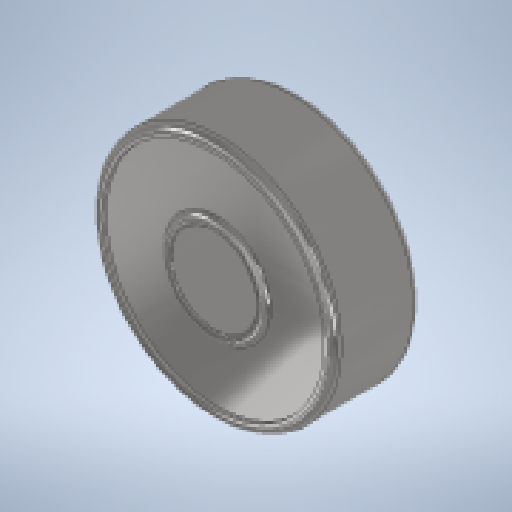
# Autodesk Inventor part: Bearing_small
Saved by Autodesk Inventor 2024 (Build 280153000, 153)
## iProperties
Created: 2025-02-20
Part Number: Bearing_small
Material: 一般
Document SubType Name: Modeling
Designer: tanoue_kota
Density: 1 g/cm^3
Appearance: 鋼 - つや出し
Author: tanoue_kota
Autodesk Inventor part; units mm, degrees
ref_plane "YZ Plane" through (0, 0, 0) normal (1, 0, 0) x (0, 1, 0)
ref_plane "XZ Plane" through (0, 0, 0) normal (0, 1, 0) x (-1, 0, 0)
ref_plane "XY Plane" through (0, 0, 0) normal (0, 0, 1) x (1, 0, 0)
sketch "スケッチ1" plane through (0, 0, 0) normal (0, 0, 1) x (1, 0, 0)
  circle A0 centre (0, 0) radius 8.5
  circle A1 centre (0, 0) radius 3
  dimension "d0" = 17
  dimension "d1" = 6
  constraints: 2 centre point, 2 coincident
  measures "d0" diameter of A0
  measures "d1" diameter of A1
extrude "押し出し1" add sketch "スケッチ1" along normal blind 3
sketch "スケッチ2" plane through (0, 0, 3) normal (0, 0, 1) x (1, 0, 0)
  circle A0 centre (0, 0) radius 7.75
  circle A1 centre (0, 0) radius 3.75
  circle A2 centre (0, 0) radius 8.5 projected
  circle A3 centre (0, 0) radius 3 projected
  dimension "d4" = 0.75
  dimension "d5" = 0.75
  constraints: 2 centre point, 2 coincident
  measures "d4" radial gap between concentric circles of A2 A0
  measures "d5" radial gap between concentric circles of A3 A1
extrude "押し出し2" cut sketch "スケッチ2" against normal blind 0.3 contours A0
mirror "ミラー1" about plane through (0, 0, 0) normal (0, 0, -1) of "押し出し1", "押し出し2"
fillet "フィレット1" radius 0.5 2 edges at (-8.5, 0, -3) (-8.5, 0, 3)
fillet "フィレット2" radius 0.1 4 edges at (-3, 0, -3) (-3, 0, 3) (-3.75, 0, -3) (-3.75, 0, 3)
